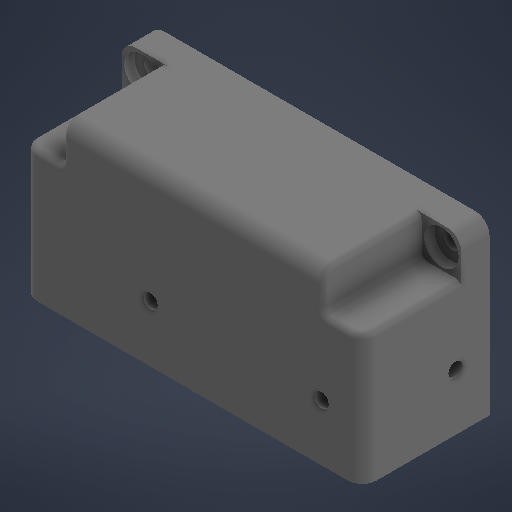
# Autodesk Inventor part: PCB_Housing_01_004
Saved by Autodesk Inventor 2026.2 (Build 302298000, 298)
## iProperties
Created: 2026-02-05
Part Number: PCB_Housing_01_004
Material: Generic
Document SubType Name: Modeling
Designer: vckot
Density: 1 g/cm^3
Appearance: Gray
Author: vckot
Autodesk Inventor part; units mm, degrees
ref_plane "YZ Plane" through (0, 0, 0) normal (1, 0, 0) x (0, 1, 0)
ref_plane "XZ Plane" through (0, 0, 0) normal (0, 1, 0) x (-1, 0, 0)
ref_plane "XY Plane" through (0, 0, 0) normal (0, 0, 1) x (1, 0, 0)
sketch "Sketch1" plane through (0, 0, 0) normal (0, 1, 0) x (-1, 0, 0)
  line L0 (-60, 60) -> (60, 60)
  line L1 (60, 60) -> (60, -60)
  line L2 (60, -60) -> (-60, -60)
  line L3 (-60, -60) -> (-60, 60)
  line L4 (-60, 60) -> (60, -60) construction
  line L5 (60, 60) -> (-60, -60) construction
  point P0 (0, 0)
  dimension "d0" = 120
  dimension "d1" = 120
  constraints: 12 end point, 2 midpoint, 2 parallel, 1 horizontal, 1 perpendicular
  measures "d0" distance of L0.end L1.end
  measures "d1" distance of L1.end L2.end
extrude "Extrusion1" add sketch "Sketch1" along normal blind 60
fillet "Fillet1" radius 5 7 edges at (0, 60, 60) (-60, 60, 0) (-60, 30, 60) (60, 30, 60) (60, 30, -60) (0, 60, -60) (-60, 30, -60)
shell "Shell1" thickness 4 removed faces 1 at (18.3333, 0, 20)
sketch "Sketch6" plane through (-55, 0, 60) normal (0, 0, 1) x (1, 0, 0)
  circle A0 centre (40.275, 20) radius 2.125 projected
  circle A1 centre (100.71, 19.949) radius 1.625 projected
  line L0 (0, 0) -> (110, 0) projected
  circle A2 centre (40.275, 20) radius 2.525
  circle A3 centre (100.71, 19.949) radius 2.525
  point P0 (55, 0)
  dimension "d32" = 20
  dimension "d33" = 19.949
  dimension "d34" = 5.05
  dimension "d35" = 5.05
  constraints: 2 centre point, 2 coincident
  measures "d32" distance from line of L0 A0.centre
  measures "d33" distance from line of L0 A1.centre
  measures "d34" diameter of A2
  measures "d35" diameter of A3
extrude "Extrusion3" cut sketch "Sketch6" against normal blind 10 contours A0 | A1 | A2 | A3
sketch "Sketch7" plane through (60, 0, 55) normal (1, 0, 0) x (0, 0, -1)
  circle A0 centre (28, 19.949) radius 1.57 projected
  circle A1 centre (28, 19.949) radius 2.525
  point P0 (55, 0)
  dimension "d38" = 5.05
  constraints: 1 centre point, 1 coincident
  measures "d38" diameter of A1
extrude "Extrusion4" cut sketch "Sketch7" against normal blind 10 contours A0 | A1
sketch "Sketch8" plane through (0, 60, 0) normal (0, 1, 0) x (1, 0, 0)
  line L0 (36.5435, 24.779) -> (13.5565, 24.779) projected
  line L1 (36.5435, 24.779) -> (36.5435, 38.241) projected
  line L2 (36.5435, 38.241) -> (13.5565, 38.241) projected
  line L3 (13.5565, 38.241) -> (13.5565, 24.779) projected
  line L4 (13.5565, 31.51) -> (36.5435, 31.51) construction
  line L5 (8.5565, 19.779) -> (41.5435, 19.779)
  line L6 (41.5435, 19.779) -> (41.5435, 43.241)
  line L7 (41.5435, 43.241) -> (8.5565, 43.241)
  line L8 (8.5565, 43.241) -> (8.5565, 19.779)
  line L9 (8.5565, 19.779) -> (41.5435, 43.241) construction
  line L10 (41.5435, 19.779) -> (8.5565, 43.241) construction
  line L11 (13.5565, 26.779) -> (36.5435, 26.779)
  line L12 (36.5435, 26.779) -> (36.5435, 36.241)
  line L13 (36.5435, 36.241) -> (13.5565, 36.241)
  line L14 (13.5565, 36.241) -> (13.5565, 26.779)
  line L15 (13.5565, 26.779) -> (36.5435, 36.241) construction
  line L16 (36.5435, 26.779) -> (13.5565, 36.241) construction
  line L17 (13.5565, 38.241) -> (13.5565, 24.779) projected
  line L18 (36.5435, 24.779) -> (36.5435, 38.241) projected
  line L19 (13.5565, 26.779) -> (36.5435, 26.779)
  line L20 (36.5435, 26.779) -> (36.5435, 36.241)
  line L21 (36.5435, 36.241) -> (13.5565, 36.241)
  line L22 (13.5565, 36.241) -> (13.5565, 26.779)
  line L23 (13.5565, 26.779) -> (36.5435, 36.241) construction
  line L24 (36.5435, 26.779) -> (13.5565, 36.241) construction
  point P0 (0, 0)
  point P1 (25.05, 31.51)
  dimension "d41" = 5
  dimension "d42" = 5
  dimension "d43" = 2
  constraints: 38 end point, 9 midpoint, 6 parallel, 3 horizontal, 3 perpendicular, 1 point on line
  measures "d41" distance from line of L7 L1.end
  measures "d42" distance from line of L6 L1.end
  measures "d43" distance from line of L0.start L11
extrude "Extrusion5" add sketch "Sketch8" against normal blind 9 contours L0 L3 L11 L1 | L11 L3 L13 L1 | L13 L3 L2 L1 | L8 L7 L6 L5
sketch "Sketch9" plane through (0, 60, 0) normal (0, 1, 0) x (1, 0, 0)
  line L0 (36.5435, 38.241) -> (13.5565, 38.241) projected
  line L1 (13.5565, 38.241) -> (13.5565, 24.779) projected
  line L2 (36.5435, 24.779) -> (13.5565, 24.779) projected
  line L3 (36.5435, 24.779) -> (36.5435, 38.241) projected
  point P0 (0, 0)
extrude "Extrusion6" cut sketch "Sketch9" against normal blind 5
sketch "Sketch10" plane through (0, 60, 0) normal (0, 1, 0) x (1, 0, 0)
  line L0 (36.5435, 36.241) -> (13.5565, 36.241) projected
  line L1 (13.5565, 26.779) -> (36.5435, 26.779) projected
  line L2 (13.5565, 24.779) -> (13.5565, 38.241) projected
  line L3 (36.5435, 24.779) -> (36.5435, 38.241) projected
  point P0 (0, 0)
extrude "Extrusion7" cut sketch "Sketch10" against normal blind 9
thicken "Thicken1" operation add thickness 0.25 both sides no extend neighbours yes toward (0, 0, -1) faces at (28.8812, 58.3333, -38.241) (13.5565, 58.3333, -29.933) (13.5565, 53.6667, -33.087) (21.2188, 58.3333, -24.779) (36.5435, 58.3333, -29.933) (36.5435, 53.6667, -29.933)
sketch "Sketch11" plane through (0, 60, 0) normal (0, 1, 0) x (1, 0, 0)
  arc A0 (-19.95, 40.8568) -> (-19.95, 44.1432) centre (-17.5, 42.5) ccw construction
  arc A1 (-26.45, 40.8568) -> (-26.45, 44.1432) centre (-24, 42.5) ccw construction
  line L0 (-24, 42.5) -> (-17.5, 42.5) construction
  line L1 (-29, 37.5) -> (-12.5, 37.5)
  line L2 (-12.5, 37.5) -> (-12.5, 47.5)
  line L3 (-12.5, 47.5) -> (-29, 47.5)
  line L4 (-29, 47.5) -> (-29, 37.5)
  line L5 (-29, 37.5) -> (-12.5, 47.5)
  line L6 (-12.5, 37.5) -> (-29, 47.5)
  circle A2 centre (-24, 42.5) radius 2.95
  circle A3 centre (-17.5, 42.5) radius 2.95
  circle A4 centre (-24, 42.5) radius 1.95
  circle A5 centre (-17.5, 42.5) radius 1.95
  circle A6 centre (-25.27, 42.5) radius 0.5 construction
  circle A7 centre (-22.73, 42.5) radius 0.5 construction
  point P0 (0, 0)
  point P1 (-20.75, 42.5)
  point P2 (-21.0558, 42.6853)
  point P3 (-20.4442, 42.6853)
  point P4 (-20.4442, 42.3146)
  point P5 (-21.0558, 42.3146)
  dimension "d52" = 5
  dimension "d53" = 5
  dimension "d54" = 5.9
  dimension "d55" = 5.9
  dimension "d56" = 1
  dimension "d57" = 1
  constraints: 14 end point, 4 centre point, 4 coincident, 3 midpoint, 2 horizontal, 2 parallel, 1 perpendicular
  measures "d52" distance from line of L2 L0.end
  measures "d53" distance from line of L3 L0.end
  measures "d54" diameter of A2
  measures "d55" diameter of A3
  measures "d56" radial gap between concentric circles of A1 A4
  measures "d57" radial gap between concentric circles of A0 A5
extrude "Extrusion8" add sketch "Sketch11" against normal blind 7
sketch "Sketch12" plane through (0, 60, 0) normal (0, 1, 0) x (1, 0, 0)
  circle A0 centre (-24, 42.5) radius 2.95
  circle A1 centre (-17.5, 42.5) radius 2.95
  circle A2 centre (-24, 42.5) radius 1.95
  circle A3 centre (-17.5, 42.5) radius 1.95
  point P0 (0, 0)
  dimension "d60" = 3.9
  dimension "d61" = 3.9
  constraints: 4 centre point, 4 coincident
  measures "d60" diameter of A2
  measures "d61" diameter of A3
extrude "Extrusion9" cut sketch "Sketch12" against normal blind 4 contours A0 | A1 | A2 | A3
extrude "Extrusion10" cut sketch "Sketch12" against normal through all contours A2 | A3
thicken "Thicken2" operation add thickness 0.25 both sides no extend neighbours yes toward (0.9967573, 0, 0.0804666) faces at (-14.5596, 57.3333, -42.2626)
thicken "Thicken3" operation add thickness 0.25 both sides no extend neighbours yes toward (0.9967573, 0, 0.0804666) faces at (-21.0596, 57.3333, -42.2626)
sketch "Sketch13" plane through (0, 60, 0) normal (0, 1, 0) x (1, 0, 0)
  line L0 (-50, -9) -> (-26, -9)
  line L1 (-26, -9) -> (-26, 33)
  line L2 (-26, 33) -> (-50, 33)
  line L3 (-50, 33) -> (-50, -9)
  line L4 (-60, 55) -> (-60, -55) projected
  line L5 (55, 60) -> (-55, 60) projected
  line L6 (-52.5, -11.5) -> (-23.5, -11.5)
  line L7 (-23.5, -11.5) -> (-23.5, 35.5)
  line L8 (-23.5, 35.5) -> (-52.5, 35.5)
  line L9 (-52.5, 35.5) -> (-52.5, -11.5)
  point P0 (0, 0)
  point P1 (-38, 33)
  point P2 (-50, 12)
  dimension "d70" = 42
  dimension "d71" = 24
  dimension "d72" = 22
  dimension "d73" = 48
  dimension "d74" = 2.5
  dimension "d75" = 2.5
  dimension "d76" = 2.5
  dimension "d77" = 2.5
  constraints: 16 end point, 4 parallel, 2 horizontal, 2 midpoint, 2 perpendicular
  measures "d70" distance of L0.end L1.end
  measures "d71" distance of L1.end L2.end
  measures "d72" distance from line of L4 point (-38, 33)
  measures "d73" distance from line of L5 point (-50, 12)
  measures "d74" distance between parallel lines of L8 L2
  measures "d75" distance between parallel lines of L9 L3
  measures "d76" distance between parallel lines of L0 L6
  measures "d77" distance between parallel lines of L1 L7
extrude "Extrusion11" add sketch "Sketch13" against normal blind 15 contours L3 L2 L1 L0 | L9 L8 L7 L6
extrude "Extrusion12" cut sketch "Sketch13" against normal blind 12.5 contours L3 L2 L1 L0
sketch "Sketch14" plane through (-26, 60, 9) normal (0, 0, -1) x (-1, 0, 0)
  line L0 (24, 0) -> (24, -12.5) projected
  line L1 (0, 0) -> (0, -12.5) projected
  line L2 (24, -12.5) -> (0, -12.5)
  line L3 (0, -12.5) -> (0, -3)
  line L4 (0, -3) -> (24, -3)
  line L5 (24, -3) -> (24, -12.5)
  point P0 (-26, -60)
  point P1 (12, -3)
  point P2 (24, -3)
  dimension "d82" = 9.5
  constraints: 8 end point, 2 parallel, 1 horizontal, 1 midpoint, 1 perpendicular, 1 point on line
  measures "d82" distance from line of L2 point (12, -3)
extrude "Extrusion13" cut sketch "Sketch14" against normal up to surface (2.5 mm away)
sketch "Sketch15" plane through (0, 60, 0) normal (0, 1, 0) x (1, 0, 0)
  line L0 (15.5683, 6.4388) -> (15.5683, 26.9695) construction
  line L1 (15.5683, 26.9695) -> (39.2414, 26.9695) construction
  line L2 (39.2414, 26.9695) -> (39.2414, 6.4388) construction
  line L3 (39.2414, 6.4388) -> (15.5683, 6.4388) construction
  line L4 (60, -55) -> (60, 55) projected
  spline S0 degree 2 poles (16.3938, 11.3722) (16.7992, 11.7182) (17.9856, 12.1038) (18.7468, 12.1038) knots 0 0 0 1 2 2 2
  spline S1 degree 2 poles (18.7468, 12.1038) (19.4883, 12.1038) (20.6896, 11.7281) (21.0949, 11.3722) knots 0 0 0 1 2 2 2
  spline S2 degree 2 poles (21.0949, 11.3722) (21.52, 10.9965) (21.9254, 10.0029) (21.9254, 9.4048) knots 0 0 0 1 2 2 2
  spline S3 degree 2 poles (21.9254, 9.4048) (21.9254, 8.7869) (21.5052, 7.7982) (21.0949, 7.4374) knots 0 0 0 1 2 2 2
  spline S4 degree 2 poles (21.0949, 7.4374) (20.6896, 7.0864) (19.4982, 6.7107) (18.7468, 6.7107) knots 0 0 0 1 2 2 2
  spline S5 degree 2 poles (18.7468, 6.7107) (17.9806, 6.7107) (16.814, 7.0913) (16.3938, 7.4423) knots 0 0 0 1 2 2 2
  spline S6 degree 2 poles (16.3938, 7.4423) (15.9885, 7.7982) (15.5683, 8.7918) (15.5683, 9.4048) knots 0 0 0 1 2 2 2
  spline S7 degree 2 poles (15.5683, 9.4048) (15.5683, 10.0276) (16.0033, 11.0262) (16.3938, 11.3722) knots 0 0 0 1 2 2 2
  spline S8 degree 2 poles (18.7468, 11.2585) (18.1438, 11.2585) (17.2095, 10.9965) (16.903, 10.7592) knots 0 0 0 1 2 2 2
  spline S9 degree 2 poles (16.903, 10.7592) (16.5866, 10.517) (16.2703, 9.8349) (16.2703, 9.4097) knots 0 0 0 1 2 2 2
  spline S10 degree 2 poles (16.2703, 9.4097) (16.2703, 8.9698) (16.5767, 8.3074) (16.903, 8.0553) knots 0 0 0 1 2 2 2
  spline S11 degree 2 poles (16.903, 8.0553) (17.2144, 7.8131) (18.1537, 7.556) (18.7468, 7.556) knots 0 0 0 1 2 2 2
  spline S12 degree 2 poles (18.7468, 7.556) (19.9481, 7.556) (21.2234, 8.5644) (21.2234, 9.4097) knots 0 0 0 1 2 2 2
  spline S13 degree 2 poles (21.2234, 9.4097) (21.2234, 10.255) (19.9481, 11.2585) (18.7468, 11.2585) knots 0 0 0 1 2 2 2
  line L5 (21.7968, 17.3585) -> (21.7968, 16.449)
  line L6 (21.7968, 16.449) -> (16.5372, 13.7499)
  line L7 (16.5372, 13.7499) -> (21.7968, 13.7499)
  line L8 (21.7968, 13.7499) -> (21.7968, 12.9936)
  line L9 (21.7968, 12.9936) -> (15.6968, 12.9936)
  line L10 (15.6968, 12.9936) -> (15.6968, 14.1454)
  line L11 (15.6968, 14.1454) -> (20.5264, 16.6022)
  line L12 (20.5264, 16.6022) -> (15.6968, 16.6022)
  line L13 (15.6968, 16.6022) -> (15.6968, 17.3585)
  line L14 (15.6968, 17.3585) -> (21.7968, 17.3585)
  spline S14 degree 2 poles (26.4373, 11.3722) (26.8427, 11.7182) (28.0291, 12.1038) (28.7903, 12.1038) knots 0 0 0 1 2 2 2
  spline S15 degree 2 poles (28.7903, 12.1038) (29.5318, 12.1038) (30.733, 11.7281) (31.1384, 11.3722) knots 0 0 0 1 2 2 2
  spline S16 degree 2 poles (31.1384, 11.3722) (31.5635, 10.9965) (31.9689, 10.0029) (31.9689, 9.4048) knots 0 0 0 1 2 2 2
  spline S17 degree 2 poles (31.9689, 9.4048) (31.9689, 8.7869) (31.5487, 7.7982) (31.1384, 7.4374) knots 0 0 0 1 2 2 2
  spline S18 degree 2 poles (31.1384, 7.4374) (30.733, 7.0864) (29.5417, 6.7107) (28.7903, 6.7107) knots 0 0 0 1 2 2 2
  spline S19 degree 2 poles (28.7903, 6.7107) (28.0241, 6.7107) (26.8575, 7.0913) (26.4373, 7.4423) knots 0 0 0 1 2 2 2
  spline S20 degree 2 poles (26.4373, 7.4423) (26.032, 7.7982) (25.6118, 8.7918) (25.6118, 9.4048) knots 0 0 0 1 2 2 2
  spline S21 degree 2 poles (25.6118, 9.4048) (25.6118, 10.0276) (26.0468, 11.0262) (26.4373, 11.3722) knots 0 0 0 1 2 2 2
  spline S22 degree 2 poles (28.7903, 11.2585) (28.1873, 11.2585) (27.253, 10.9965) (26.9465, 10.7592) knots 0 0 0 1 2 2 2
  spline S23 degree 2 poles (26.9465, 10.7592) (26.6301, 10.517) (26.3138, 9.8349) (26.3138, 9.4097) knots 0 0 0 1 2 2 2
  spline S24 degree 2 poles (26.3138, 9.4097) (26.3138, 8.9698) (26.6202, 8.3074) (26.9465, 8.0553) knots 0 0 0 1 2 2 2
  spline S25 degree 2 poles (26.9465, 8.0553) (27.2579, 7.8131) (28.1971, 7.556) (28.7903, 7.556) knots 0 0 0 1 2 2 2
  spline S26 degree 2 poles (28.7903, 7.556) (29.9915, 7.556) (31.2669, 8.5644) (31.2669, 9.4097) knots 0 0 0 1 2 2 2
  spline S27 degree 2 poles (31.2669, 9.4097) (31.2669, 10.255) (29.9915, 11.2585) (28.7903, 11.2585) knots 0 0 0 1 2 2 2
  line L15 (26.4621, 16.6417) -> (26.4621, 13.8043)
  line L16 (26.4621, 13.8043) -> (28.1823, 13.8043)
  line L17 (28.1823, 13.8043) -> (28.1823, 16.5231)
  line L18 (28.1823, 16.5231) -> (28.904, 16.5231)
  line L19 (28.904, 16.5231) -> (28.904, 13.8043)
  line L20 (28.904, 13.8043) -> (31.8403, 13.8043)
  line L21 (31.8403, 13.8043) -> (31.8403, 12.9936)
  line L22 (31.8403, 12.9936) -> (25.7403, 12.9936)
  line L23 (25.7403, 12.9936) -> (25.7403, 16.6417)
  line L24 (25.7403, 16.6417) -> (26.4621, 16.6417)
  line L25 (26.4621, 21.0165) -> (26.4621, 18.1791)
  line L26 (26.4621, 18.1791) -> (28.1823, 18.1791)
  line L27 (28.1823, 18.1791) -> (28.1823, 20.8979)
  line L28 (28.1823, 20.8979) -> (28.904, 20.8979)
  line L29 (28.904, 20.8979) -> (28.904, 18.1791)
  line L30 (28.904, 18.1791) -> (31.8403, 18.1791)
  line L31 (31.8403, 18.1791) -> (31.8403, 17.3684)
  line L32 (31.8403, 17.3684) -> (25.7403, 17.3684)
  line L33 (25.7403, 17.3684) -> (25.7403, 21.0165)
  line L34 (25.7403, 21.0165) -> (26.4621, 21.0165)
  point P0 (0, 0)
  constraints: 2 other
extrude "Extrusion14" cut sketch "Sketch15" against normal blind 2
sketch "Sketch16" plane through (0, 47.5, 0) normal (0, 1, 0) x (1, 0, 0)
  line L0 (-50, 33) -> (-26, 33) projected
  line L1 (-26, -9) -> (-50, -9) projected
  line L2 (-45, 33) -> (-31, 33)
  line L3 (-31, 33) -> (-31, -9)
  line L4 (-31, -9) -> (-45, -9)
  line L5 (-45, -9) -> (-45, 33)
  line L6 (-50, -9) -> (-50, 33) projected
  line L7 (-26, 33) -> (-26, -9) projected
  point P0 (0, 0)
  dimension "d88" = 5
  dimension "d89" = 5
  constraints: 8 end point, 2 parallel, 2 point on line, 1 horizontal, 1 perpendicular
  measures "d88" distance between parallel lines of L6 L5
  measures "d89" distance between parallel lines of L7 L3
extrude "Extrusion15" cut sketch "Sketch16" against normal through all contours L0 L3 L1 L5
delete faces "Delete Face1" heal yes whole lump no faces at (-40.3333, 46.6667, 9)
sketch "Sketch17" plane through (-50, 47.5, -33) normal (0, 1, 0) x (1, 0, 0)
  circle A0 centre (2, -40) radius 1.1 projected
  circle A1 centre (2, -2) radius 1.1 projected
  circle A2 centre (22, -2) radius 1.1 projected
  circle A3 centre (22, -40) radius 1.1 projected
  point P0 (50, -33)
extrude "Extrusion16" cut sketch "Sketch17" against normal through all
fillet "Fillet2" radius 5 3 edges at (58.5355, 58.5355, -58.5355) (58.5355, 58.5355, 58.5355) (60, 60, 0)
sketch "Sketch18" plane through (56, 0, -55) normal (-1, 0, 0) x (0, 0, 1)
  line L0 (2.5, 25.4) -> (2.5, 56) projected
  line L1 (44.0432, 56) -> (2.5, 56) projected
  line L2 (7.44, 25.4) -> (7.44, 51) projected
  line L3 (7.44, 51) -> (39.0432, 51) projected
  line L4 (39.0432, 51) -> (39.0432, 39.5) projected
  line L5 (39.0432, 39.5) -> (27.36, 39.5) projected
  line L6 (39.0432, 51) -> (39.0432, 39.5) projected
  line L7 (39.0432, 39.5) -> (27.36, 39.5) projected
  line L8 (27.36, 39.5) -> (27.36, 25.4) projected
  line L9 (27.36, 25.4) -> (32.3, 25.4) projected
  line L10 (32.3, 25.4) -> (32.3, 34.5) projected
  line L11 (32.3, 34.5) -> (44.0432, 34.5) projected
  line L12 (44.0432, 34.5) -> (44.0432, 56) projected
  line L13 (44.0432, 56) -> (2.5, 56) projected
  line L14 (2.5, 25.4) -> (2.5, 56) projected
  line L15 (2.5, 25.4) -> (7.44, 25.4) projected
  line L16 (7.44, 25.4) -> (7.44, 51) projected
  line L17 (7.44, 51) -> (39.0432, 51) projected
  line L18 (2.5, 25.4) -> (32.3, 25.4) projected
  line L19 (-1, 0) -> (-1, 55) projected
  line L20 (2.5, 56) -> (-1, 56)
  line L21 (-1, 56) -> (-1, 25.4)
  line L22 (-1, 25.4) -> (2.5, 25.4)
  line L23 (2.5, 25.4) -> (2.5, 56)
  point P0 (55, 0)
  constraints: 8 end point, 2 parallel, 1 horizontal, 1 perpendicular, 1 point on line
extrude "Extrusion17" add sketch "Sketch18" along normal blind 5
sketch "Sketch19" plane through (51, 0, -55) normal (-1, 0, 0) x (0, 0, 1)
  line L0 (2.5, 25.4) -> (2.5, 56) projected
  line L1 (7.44, 51) -> (39.0432, 51) projected
  line L2 (7.44, 25.4) -> (7.44, 51) projected
  line L3 (-1, 25.4) -> (32.3, 25.4) projected
  line L4 (27.36, 39.5) -> (27.36, 25.4) projected
  line L5 (39.0432, 39.5) -> (27.36, 39.5) projected
  line L6 (39.0432, 51) -> (39.0432, 39.5) projected
  line L7 (44.0432, 34.5) -> (44.0432, 56) projected
  line L8 (44.0432, 34.5) -> (32.3, 34.5) projected
  line L9 (32.3, 25.4) -> (32.3, 34.5) projected
  line L10 (2.5, 25.4) -> (32.3, 25.4) projected
  line L11 (-1, 25.4) -> (-1, 55) projected
  line L12 (2.5, 56) -> (44.0432, 56) projected
  line L13 (2.5, 56) -> (-1, 56)
  line L14 (-1, 56) -> (-1, 55)
  point P0 (55, 0)
  constraints: 4 end point, 1 horizontal, 1 perpendicular
extrude "Extrusion18" add sketch "Sketch19" along normal blind 7.5 contours L3 L11 L14 L13 L0 | L0 L12 L7 L8 L9 L3 L4 L5 L6 L1 L2
sketch "Sketch20" plane through (55, 0, -60) normal (0, 0, -1) x (-1, 0, 0)
  circle A0 centre (7.2, 43.8735) radius 2.5 projected
  circle A1 centre (7.2, 43.8735) radius 2.525
  point P0 (55, 0)
  dimension "d99" = 5.05
  constraints: 1 centre point, 1 coincident
  measures "d99" diameter of A1
extrude "Extrusion19" cut sketch "Sketch20" against normal blind 100 contours A0 | A1
sketch "Sketch21" plane through (60, 0, 55) normal (1, 0, 0) x (0, 0, -1)
  line L0 (0, 0) -> (110, 0) projected
  line L1 (115, 60) -> (40, 60)
  line L2 (40, 60) -> (40, 0)
  line L3 (40, 0) -> (115, 0)
  line L4 (115, 0) -> (115, 60)
  point P0 (55, 0)
  dimension "d102" = 75
  dimension "d103" = 60
  constraints: 8 end point, 2 parallel, 1 horizontal, 1 perpendicular, 1 point on line
  measures "d102" distance of L1.start L1.end
  measures "d103" distance of L3.end L1.start
extrude "Extrusion20" cut sketch "Sketch21" against normal through all
sketch "Sketch22" plane through (60, 0, 15) normal (0, 0, -1) x (-1, 0, 0)
  arc A0 (5, 60) -> (0, 55) centre (5, 55) ccw projected
  arc A1 (120, 55) -> (115, 60) centre (115, 55) ccw projected
  line L0 (0, 60) -> (17, 60)
  line L1 (17, 60) -> (17, 43)
  line L2 (17, 43) -> (0, 43)
  line L3 (0, 43) -> (0, 60)
  line L4 (120, 60) -> (103, 60)
  line L5 (103, 60) -> (103, 43)
  line L6 (103, 43) -> (120, 43)
  line L7 (120, 43) -> (120, 60)
  line L8 (5, 60) -> (115, 60) projected
  line L9 (0, 0) -> (0, 55) projected
  line L10 (120, 55) -> (120, 0) projected
  line L11 (0, 60) -> (14, 60)
  line L12 (14, 60) -> (14, 46)
  line L13 (14, 46) -> (0, 46)
  line L14 (0, 46) -> (0, 60)
  line L15 (120, 60) -> (106, 60)
  line L16 (106, 60) -> (106, 46)
  line L17 (106, 46) -> (120, 46)
  line L18 (120, 46) -> (120, 60)
  point P0 (60, 0)
  point P1 (14, 60)
  dimension "d106" = 17
  dimension "d107" = 17
  dimension "d108" = 17
  dimension "d109" = 17
  dimension "d110" = 14
  dimension "d111" = 14
  dimension "d112" = 14
  dimension "d113" = 14
  constraints: 32 end point, 8 parallel, 4 horizontal, 4 perpendicular, 3 collinear, 1 point on line
  measures "d106" distance of L1.end L2.end
  measures "d107" distance of L0.end L1.end
  measures "d108" distance of L6.end L5.end
  measures "d109" distance of L5.end L4.end
  measures "d110" distance of L12.end L13.end
  measures "d111" distance of L11.end L12.end
  measures "d112" distance of L17.end L16.end
  measures "d113" distance of L16.end L15.end
extrude "Extrusion21" add sketch "Sketch22" against normal through all contours L0 L1 L2 L3 L13 L12 | L7 L6 L5 L4 L16 L17
extrude "Extrusion22" cut sketch "Sketch22" against normal through all contours L0 L12 L13 L3 A0 | L7 L17 L16 L4 A1
extrude "Extrusion23" add sketch "Sketch22" against normal blind 10 contours L0 L12 L13 L3 A0 | L7 L17 L16 L4 A1
fillet "Fillet4" radius 2 16 edges at (46, 58.5355, 58.5355) (46, 50.5, 60) (46, 60, 40) (58.5355, 46, 58.5355) (50.5, 46, 60) (60, 46, 40) (46, 46, 42.5) (-46, 58.5355, 58.5355) (-46, 50.5, 60) (-46, 60, 40) (-46, 46, 42.5) (-58.5355, 46, 58.5355) (-50.5, 46, 60) (-60, 46, 40) (-43, 43, 35.5) (43, 43, 35.5)
sketch "Sketch23" plane through (60, 0, 25) normal (0, 0, 1) x (1, 0, 0)
  line L0 (0, 44) -> (0, 55) projected
  line L1 (-5, 60) -> (-16, 60) projected
  line L2 (-120, 55) -> (-120, 44) projected
  line L3 (-104, 60) -> (-115, 60) projected
  point P0 (-60, 0)
  point P1 (-113, 53)
  point P2 (-7, 53)
  dimension "d122" = 7
  dimension "d123" = 7
  dimension "d124" = 7
  dimension "d125" = 7
  measures "d122" distance from line of L0 point (-7, 53)
  measures "d123" distance from line of L1 point (-7, 53)
  measures "d124" distance from line of L2 point (-113, 53)
  measures "d125" distance from line of L3 point (-113, 53)
hole "Hole4" at (-53, 53, 25) at (53, 53, 25) direction (0, 0, -1) diameter 5.5 end through all counterbore diameter 12.24 counterbore depth 3.65 clearance for "Hex Head Cap Screw" size "M5" standard "Ansi Metric M Profile"
sketch "Sketch24" plane through (0, 0, 0) normal (0, -1, 0) x (1, 0, 0)
  arc A0 (60, 55) -> (55, 60) centre (55, 55) ccw projected
  arc A1 (-55, 60) -> (-60, 55) centre (-55, 55) ccw projected
  line L0 (-60, 60) -> (-46, 60)
  line L1 (-46, 60) -> (-46, 46)
  line L2 (-46, 46) -> (-60, 46)
  line L3 (-60, 46) -> (-60, 60)
  line L4 (60, 60) -> (46, 60)
  line L5 (46, 60) -> (46, 46)
  line L6 (46, 46) -> (60, 46)
  line L7 (60, 46) -> (60, 60)
  line L8 (-60, 15) -> (-60, 55) projected
  line L9 (-55, 60) -> (55, 60) projected
  line L10 (60, 55) -> (60, 15) projected
  point P0 (0, 0)
  point P1 (60, 55)
  dimension "d133" = 14
  dimension "d134" = 14
  dimension "d135" = 14
  dimension "d136" = 14
  constraints: 16 end point, 4 parallel, 3 collinear, 2 horizontal, 2 perpendicular, 1 point on line
  measures "d133" distance of L1.end L2.end
  measures "d134" distance of L0.end L1.end
  measures "d135" distance of L6.end L5.end
  measures "d136" distance of L5.end L4.end
extrude "Extrusion24" add sketch "Sketch24" against normal blind 10 contours L7 L6 L5 L4 A0 | L0 L1 L2 L3 A1
sketch "Sketch25" plane through (0, 0, 0) normal (0, -1, 0) x (1, 0, 0)
  line L0 (-60, 15) -> (-60, 55) projected
  line L1 (-55, 60) -> (55, 60) projected
  line L2 (60, 55) -> (60, 15) projected
  point P0 (0, 0)
  point P1 (-53, 53)
  point P2 (53, 53)
  dimension "d146" = 7
  dimension "d147" = 7
  dimension "d148" = 7
  dimension "d149" = 7
  measures "d146" distance from line of L0 point (-53, 53)
  measures "d147" distance from line of L1 point (-53, 53)
  measures "d148" distance from line of L1 point (53, 53)
  measures "d149" distance from line of L2 point (53, 53)
hole "Hole5" at (-53, 0, 53) at (53, 0, 53) direction (0, 1, 0) diameter 6.4 depth 10 tip angle 118
body "Solid1"
